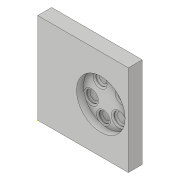
# Autodesk Inventor part: bottom support
Saved by Autodesk Inventor 2019 (Build 230136000, 136)
## iProperties
Created: 2019-10-07
Part Number: bottom support
Material: Generic
Document SubType Name: Modeling
Designer: Admin
Density: 1 g/cm^3
Appearance: Default
Author: Admin
Autodesk Inventor part; units mm, degrees
ref_plane "YZ Plane" through (0, 0, 0) normal (1, 0, 0) x (0, 1, 0)
ref_plane "XZ Plane" through (0, 0, 0) normal (0, 1, 0) x (-1, 0, 0)
ref_plane "XY Plane" through (0, 0, 0) normal (0, 0, 1) x (1, 0, 0)
sketch "Sketch1" plane through (0, 0, 0) normal (0, 0, 1) x (1, 0, 0)
  line L0 (0, 0) -> (130, 0)
  line L1 (130, 0) -> (130, 130)
  line L2 (130, 130) -> (0, 130)
  line L3 (0, 130) -> (0, 0)
  dimension "d0" = 130
  dimension "d1" = 130
  constraints: 8 end point, 2 parallel, 1 horizontal, 1 perpendicular
  measures "d0" distance of L2.end L1.end
  measures "d1" distance of L1.end L0.end
extrude "Extrusion1" add sketch "Sketch1" along normal blind 20
sketch "Sketch2" plane through (0, 0, 20) normal (0, 0, 1) x (1, 0, 0)
  line L0 (0, 0) -> (130, 0) projected
  line L1 (0, 0) -> (10, 0)
  line L2 (10, 0) -> (10, 130.175)
  line L3 (10, 130.175) -> (119.9999, 130)
  line L4 (130, 130) -> (0, 130) projected
  line L5 (119.9999, 130) -> (119.793, 0)
  line L6 (119.793, 0) -> (119.809, 10)
  line L7 (119.809, 10) -> (9.809, 10)
  line L8 (9.809, 10) -> (10, 119.9998)
  line L9 (10, 119.9998) -> (119.9998, 119.8088)
  line L10 (0, 130) -> (0, 125.4125)
  line L11 (0, 125.4125) -> (0, 60.4125)
  line L12 (0, 130) -> (0, 0) projected
  line L13 (0, 60.4125) -> (35, 60.4125)
  circle A0 centre (10, 119.9998) radius 5
  circle A1 centre (119.9998, 119.8088) radius 5
  circle A2 centre (9.809, 10) radius 5
  circle A3 centre (119.809, 10) radius 5
  line L14 (0, 60.4125) -> (30, 60.4125)
  circle A4 centre (30, 60.4125) radius 5.5
  dimension "d4" = 10
  dimension "d5" = 110
  dimension "d6" = 10
  dimension "d7" = 110
  dimension "d8" = 110
  dimension "d9" = 110
  dimension "d10" = 65
  dimension "d11" = 35
  dimension "d12" = 10
  dimension "d13" = 10
  dimension "d14" = 10
  dimension "d15" = 10
  dimension "d51" = 30
  dimension "d52" = 11
  constraints: 24 end point, 7 point on line, 5 centre point, 5 coincident, 5 perpendicular
  measures "d4" distance of L0.start L1.end
  measures "d5" distance of L2.end L3.end
  measures "d6" distance of L5.end L6.end
  measures "d7" distance of L6.end L7.end
  measures "d8" distance of L7.end L8.end
  measures "d9" distance of L8.end L9.end
  measures "d10" distance of L10.end L11.end
  measures "d11" distance of L11.end L13.end
  measures "d12" diameter of A0
  measures "d13" diameter of A1
  measures "d14" diameter of A2
  measures "d15" diameter of A3
  measures "d51" distance of L11.end L14.end
  measures "d52" diameter of A4
extrude "Extrusion2" [suppressed]
thread "Thread1" size "M10x1.5" class "6H" standard "ANSI Metric M Profile" full length
thread "Thread2" size "M10x1.5" class "6H" standard "ANSI Metric M Profile" full length
thread "Thread3" size "M10x1.5" class "6H" standard "ANSI Metric M Profile" full length
thread "Thread4" size "M10x1.5" class "6H" standard "ANSI Metric M Profile" full length
thread "Thread5" size "M10x1.5" class "6H" standard "ANSI Metric M Profile" full length
thread "Thread6" size "M10x1.5" class "6H" standard "ANSI Metric M Profile" full length
thread "Thread7" size "M10x1.5" class "6H" standard "ANSI Metric M Profile" full length
thread "Thread8" size "M10x1.5" class "6H" standard "ANSI Metric M Profile" full length
sketch "Sketch3" plane through (0, 0, 20) normal (0, 0, 1) x (1, 0, 0)
  line L0 (130, 0) -> (130, 130) projected
  line L1 (130, 65) -> (120, 65)
  line L2 (120, 65) -> (60, 65)
  circle A0 centre (90, 65) radius 30
  circle A1 centre (90, 65) radius 10
  circle A2 centre (74.6125, 52.3875) radius 9.5932
  circle A3 centre (101.6, 49.2125) radius 9.5909
  circle A4 centre (107.95, 72.1652) radius 8.4813
  circle A5 centre (74.6125, 75) radius 8.9266
  circle A6 centre (93.6625, 83.9266) radius 8.3145
  point P0 (0, 0)
  dimension "d37" = 10
  dimension "d38" = 60
  dimension "d39" = 60
  dimension "d40" = 20
  constraints: 7 centre point, 4 end point, 2 midpoint, 1 coincident, 1 horizontal, 1 point on line, 1 tangent
  measures "d37" distance of L1.start L1.end
  measures "d38" distance of L1.end L2.end
  measures "d39" diameter of A0
  measures "d40" diameter of A1
extrude "Extrusion3" cut sketch "Sketch3" against normal blind 7.5 contours A3 | A4 L2 | L2 A4 | A5 A1 | A1 A5 | A2 | A6
fillet "Fillet1" radius 5 5 edges at (65.6859, 75, 12.5) (85.348, 83.9266, 12.5) (65.0193, 52.3875, 12.5) (92.0091, 49.2125, 12.5) (99.4687, 72.1652, 12.5)
sketch "Sketch4" plane through (0, 0, 20) normal (0, 0, 1) x (1, 0, 0)
  circle A0 centre (90.4875, 65.0875) radius 31.75
  point P0 (0, 0)
  constraints: 1 centre point
extrude "Extrusion4" cut sketch "Sketch4" along normal blind 20
sketch "Sketch5" plane through (0, 0, 20) normal (0, 0, 1) x (1, 0, 0)
  point P0 (0, 0)
sketch "Sketch6" plane through (0, 0, 20) normal (0, 0, 1) x (1, 0, 0)
  circle A0 centre (90.4875, 65.0875) radius 34.8166
  point P0 (0, 0)
  constraints: 1 centre point
extrude "Extrusion5" cut sketch "Sketch6" against normal blind 10
sketch "Sketch7" plane through (90.4875, 65.0875, 10) normal (0, 0, 1) x (1, 0, 0)
  circle A0 centre (20.6375, 14.2875) radius 8.1026
  circle A1 centre (-11.1125, 19.05) radius 8.0947
  circle A2 centre (15.875, -15.875) radius 8.9803
  circle A3 centre (-23.8125, -7.9375) radius 8.5489
  circle A4 centre (-6.35, -24.8553) radius 7.9375
  point P0 (-90.4875, -65.0875)
  constraints: 5 centre point
extrude "Extrusion6" cut sketch "Sketch7" against normal blind 5
fillet "Fillet2" radius 2 10 edges at (97.3822, 49.2125, 10) (76.2, 40.2322, 10) (58.1261, 57.15, 5) (71.2803, 84.1375, 5) (103.0224, 79.375, 10) (103.0224, 79.375, 5) (58.1261, 57.15, 10) (71.2803, 84.1375, 10) (76.2, 40.2322, 5) (97.3822, 49.2125, 5)
body "Solid1"
